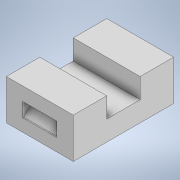
# Autodesk Inventor part: Тестовая коробка
Saved by Autodesk Inventor 2020 (Build 240168000, 168)
## iProperties
Created: 2021-04-26
Part Number: Тестовая коробка
Material: Типовые
Document SubType Name: Modeling
Designer: Антон
Density: 1 g/cm^3
Appearance: По умолчанию
Author: Антон
Autodesk Inventor part; units mm, degrees
ref_plane "YZ Plane" through (0, 0, 0) normal (1, 0, 0) x (0, 1, 0)
ref_plane "XZ Plane" through (0, 0, 0) normal (0, 1, 0) x (-1, 0, 0)
sketch "Эскиз1" plane through (0, 0, 0) normal (0, 1, 0) x (-1, 0, 0)
  line L0 (0, 0) -> (10, 0)
  line L1 (10, 0) -> (10, -15)
  line L2 (10, -15) -> (0, -15)
  line L3 (0, -15) -> (0, 0)
  dimension "d0" = 10
  dimension "d1" = 15
  constraints: 8 end point, 2 parallel, 1 horizontal, 1 perpendicular
  measures "d0" distance of L1.end L2.end
  measures "d1" distance of L0.end L1.end
extrude "Выдавливание1" add sketch "Эскиз1" along normal blind 6
sketch "Эскиз2" plane through (0, 6, 0) normal (0, 1, 0) x (1, 0, 0)
  line L0 (-10, 15) -> (-10, 0) projected
  line L1 (-10, 0) -> (-10, 5)
  line L2 (0, 0) -> (0, 15) projected
  line L3 (-10, 5) -> (0, 5)
  line L4 (0, 5) -> (0, 10)
  line L5 (0, 10) -> (-10, 10)
  line L6 (-10, 10) -> (-10, 5)
  line L7 (-10, 10) -> (-10, 15)
  line L8 (-10, 0) -> (0, 0) projected
  point P0 (0, 5)
  dimension "d4" = 5
  constraints: 12 end point, 2 collinear, 2 parallel, 2 point on line, 1 horizontal, 1 perpendicular
  measures "d4" distance between parallel lines of L8 L3
extrude "Выдавливание2" cut sketch "Эскиз2" against normal blind 3 contours L5 L2 L3 L0
sketch "Эскиз3" plane through (-10, 0, 0) normal (0, 0, 1) x (1, 0, 0)
  line L0 (2.45, 4) -> (7.55, 4)
  line L1 (7.55, 4) -> (7.55, 1.9)
  line L2 (7.55, 1.9) -> (2.45, 1.9)
  line L3 (2.45, 1.9) -> (2.45, 4)
  line L4 (2.45, 2.95) -> (0, 2.95)
  line L5 (0, 0) -> (0, 6) projected
  line L6 (7.55, 2.95) -> (10, 2.95)
  line L7 (10, 0) -> (10, 6) projected
  line L8 (5, 4) -> (5, 6)
  line L9 (10, 6) -> (0, 6) projected
  dimension "d7" = 5.1
  dimension "d8" = 2.1
  dimension "d12" = 2
  constraints: 14 end point, 4 midpoint, 3 point on line, 2 horizontal, 2 parallel, 1 collinear, 1 perpendicular
  measures "d7" distance between parallel lines of L1 L3
  measures "d8" distance between parallel lines of L2 L0
  measures "d12" distance of L8.start L8.end
extrude "Выдавливание3" cut sketch "Эскиз3" against normal blind 2.15 contours L0 L1 L2 L3
ref_plane "РабПлоскость1" through (-10, 6, -7.5) normal (0, 0, 1) x (1, 0, 0)
mirror "Зеркальное отражение1" about plane through (-10, 6, -7.5) normal (0, 0, 1) of "Выдавливание3"
chamfer "Фаска1" distance 2 angle 45 2 edges at (-5, 1.9, -2.15) (-5, 1.9, -12.85)
